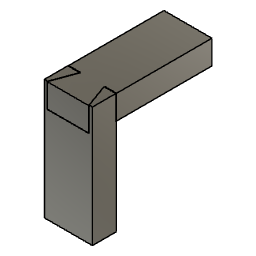
Dovetail Joint (Autodesk Fusion 360 design; units mm, degrees)
Autodesk Fusion 360 part; units mm, degrees
sketch "Base" plane through (0, 0, 0) normal (0, 0, 1) x (1, 0, 0)
  line L0 (-30, 25) -> (10, 25)
  line L1 (10, 25) -> (10, 5)
  line L2 (10, 5) -> (-30, 5)
  line L3 (-30, 5) -> (-30, 25)
  dimension "d6" = 40
  dimension "d7" = 20
  constraint horizontal L0
  constraint vertical L1
  constraint horizontal L2
  constraint vertical L3
  measures "d6" distance of L0.start L0.end
  measures "d7" distance of L0.start L2.end
extrude "Extrude1" add sketch "Base" along normal blind 100 makes body 1
sketch "Top" plane through (0, 0, 100) normal (0, 0, 1) x (-1, 0, 0)
  line L0 (30, -5) -> (-10, -5)
  line L1 (-10, -5) -> (-10, -25)
  line L2 (-10, -25) -> (30, -25)
  line L3 (30, -25) -> (30, -5)
  line L4 (30, -5) -> (-10, -5)
  line L5 (-10, -5) -> (-10, -105)
  line L6 (-10, -105) -> (30, -105)
  line L7 (30, -105) -> (30, -5)
  line L8 (-10, -25) -> (0, -25)
  line L9 (0, -25) -> (-7.2794, -5)
  line L10 (-7.2794, -5) -> (27.2794, -5)
  line L11 (27.2794, -5) -> (20, -25)
  line L12 (30, -25) -> (20, -25)
  dimension "d10" = 40
  dimension "d11" = 100
  dimension "d12" = 10
  dimension "d13" = 10
  dimension "d14" = 70
  dimension "d15" = 70
  constraint horizontal L4
  constraint vertical L5
  constraint horizontal L6
  constraint vertical L7
  constraint coincident L0.start L3.end
  constraint coincident L1.end L2.start
  constraint coincident L2 L8.end
  constraint perpendicular L5 L8
  constraint parallel L0 L10
  constraint coincident L2 L11.end
  constraint coincident L2.end L3.start
  constraint collinear L4 L10
  measures "d10" distance of L0.start L0.end
  measures "d11" distance of L0.start L6.end
  measures "d12" distance of L1.end L8.end
  measures "d13" distance of L11.end L2.end
  measures "d14" angle of L8 L9
  measures "d15" angle of L11 L12
extrude "Extrude1'" add sketch "Top" against normal blind 20 separate body contours L0 L2 L4 L9 L10 L11 | L2 L5 L6 L7 L8 L12 makes body 2 in component "Top"
combine "Combine1" operation cut target body 1 tool bodies 2 keep tools
copy_body "Body->Comp1" bodies 1 removing the originals makes body 3 in component "Bottom"
component "Top" placed x (1, 0, 0) y (0, 1, 0) z (0, 0, 1) at (0, 0, 0)
component "Bottom" placed x (1, 0, 0) y (0, 1, 0) z (0, 0, 1) at (0, 0, 0)
equation "width = 40 mm"
equation "lenght = 100 mm"
equation "thickness = 20 mm"
equation "pin = 10 mm"
equation "angle = 70 deg"
equation "d6 = width"
equation "d7 = thickness"
equation "d8 = lenght"
equation "d10 = width"
equation "d11 = lenght"
equation "d12 = pin"
equation "d13 = pin"
equation "d14 = angle"
equation "d15 = angle"
equation "d16 = -thickness"
